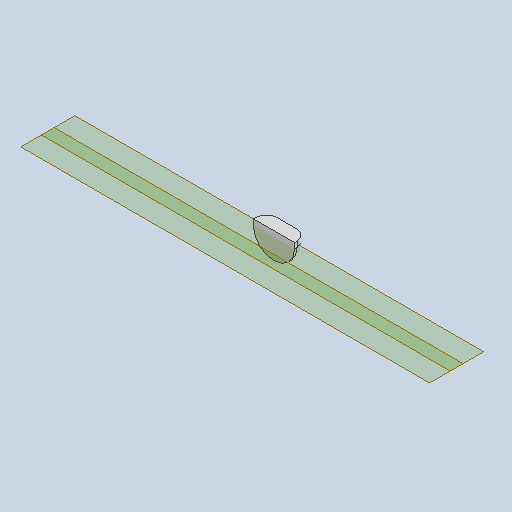
# Autodesk Inventor part: AvionicsBay
Saved by Autodesk Inventor 2025 (Build 290162000, 162)
## iProperties
Created: 2024-09-16
Part Number: AvionicsBay
Material: Generic
Document SubType Name: Modeling
Designer: Cupri
Density: 1 g/cm^3
Appearance: Default
Author: Cupri
Autodesk Inventor part; units mm, degrees
ref_plane "YZ Plane" through (0, 0, 0) normal (1, 0, 0) x (0, 1, 0)
ref_plane "XZ Plane" through (0, 0, 0) normal (0, 1, 0) x (-1, 0, 0)
ref_plane "XY Plane" through (0, 0, 0) normal (0, 0, 1) x (1, 0, 0)
ref_plane "Work Plane1" through (152.4, 0, 203.2) normal (0, -1, 0) x (1, 0, 0)
ref_plane "Work Plane2" through (-50.8, 26.2952, 0) normal (0, -1, 0) x (1, 0, 0)
ref_plane "Work Plane4" through (152.4, 0, 101.6) normal (0, -1, 0) x (1, 0, 0)
sketch "Sketch3" plane through (152.4, 0, 101.6) normal (0, -1, 0) x (1, 0, 0)
  arc A0 (0, -25.4) -> (-76.2, 50.8) centre (-76.2, -25.4) ccw
  line L0 (-127, 50.8) -> (-76.2, 50.8)
  arc A1 (0, -25.4) -> (-76.2, 50.8) centre (-76.2, -25.4) ccw
  line L1 (0, -50.8) -> (0, -25.4)
  arc A2 (-50.8, -101.6) -> (0, -50.8) centre (-50.8, -50.8) ccw
  line L2 (-152.4, -101.6) -> (-50.8, -101.6)
  line L3 (-101.6, 50.8) -> (-101.6, -101.6)
  line L4 (-165.1, -38.1) -> (-41.6, -38.1) construction
  line L5 (-103.35, -38.1) -> (0, -38.1)
  point P0 (-101.6, -38.1)
revolve "Revolution2" add sketch "Sketch3" angle 180 about axis through (50.8, 0, 152.4) along (0, 0, -1) contours L1 A2 L2 L3 L5
sketch "Sketch4" plane through (-50.8, 0, 63.5) normal (0, 1, 0) x (1, 0, 0)
  line L0 (203.2, 12.7) -> (203.2, 0) projected
  arc A0 (203.2, 12.7) -> (152.4, 63.5) centre (152.4, 12.7) ccw projected
  line L1 (152.4, 63.5) -> (50.8, 63.5) projected
  arc A1 (50.8, 63.5) -> (0, 12.7) centre (50.8, 12.7) ccw projected
  line L2 (0, 12.7) -> (0, 0) projected
  line L3 (203.2, 0) -> (0, 0) projected
  point P0 (50.8, 63.5)
ref_plane "Work Plane5" through (-50.8, 26.2952, 0) normal (0, -1, 0) x (1, 0, 0)
extrude "Extrusion2" add sketch "Sketch4" along normal up to surface (26.2952 mm away)
body "Solid2"
